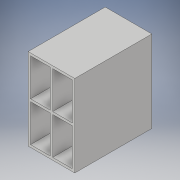
# Autodesk Inventor part: batterycart skeleton
Saved by Autodesk Inventor 2019 (Build 230136000, 136)
## iProperties
Created: 2018-12-03
Part Number: batterycart skeleton
Material: Generic
Document SubType Name: Modeling
Designer: Tiberus
Density: 1 g/cm^3
Appearance: Default
Author: Tiberus
Autodesk Inventor part; units mm, degrees
ref_plane "YZ Plane" through (0, 0, 0) normal (1, 0, 0) x (0, 1, 0)
ref_plane "XZ Plane" through (0, 0, 0) normal (0, 1, 0) x (-1, 0, 0)
ref_plane "XY Plane" through (0, 0, 0) normal (0, 0, 1) x (1, 0, 0)
sketch "Sketch1" plane through (0, 0, 0) normal (0, 0, 1) x (1, 0, 0)
  line L0 (0, 0) -> (241.3, 0)
  line L1 (241.3, 0) -> (241.3, 423.164)
  line L2 (241.3, 423.164) -> (0, 423.164)
  line L3 (0, 423.164) -> (0, 0)
  line L4 (120.65, 423.164) -> (120.65, 0) construction
  line L5 (241.3, 211.582) -> (0, 211.582) construction
  line L6 (159.3781, 211.582) -> (159.3781, 217.932) construction
  line L7 (120.65, 100.386) -> (127, 100.386) construction
  line L8 (196.0731, 0) -> (196.0731, 12.7) construction
  line L9 (142.6395, 423.164) -> (142.6395, 410.464) construction
  line L10 (127, 410.464) -> (228.6, 410.464)
  line L11 (127, 217.932) -> (228.6, 217.932)
  line L12 (228.6, 217.932) -> (228.6, 410.464)
  line L13 (241.3, 374.8885) -> (228.6, 374.8885) construction
  line L14 (174.8387, 211.582) -> (174.8387, 205.232) construction
  line L15 (127, 205.232) -> (228.6, 205.232)
  line L16 (228.6, 205.232) -> (228.6, 12.7)
  line L17 (228.6, 12.7) -> (127, 12.7)
  line L18 (127, 12.7) -> (127, 205.232)
  line L19 (127, 217.932) -> (127, 410.464)
  line L20 (81.9219, 211.582) -> (81.9219, 217.932) construction
  line L21 (114.3, 410.464) -> (12.7, 410.464)
  line L22 (114.3, 217.932) -> (12.7, 217.932)
  line L23 (12.7, 217.932) -> (12.7, 410.464)
  line L24 (66.4613, 211.582) -> (66.4613, 205.232) construction
  line L25 (114.3, 205.232) -> (12.7, 205.232)
  line L26 (12.7, 205.232) -> (12.7, 12.7)
  line L27 (12.7, 12.7) -> (114.3, 12.7)
  line L28 (114.3, 12.7) -> (114.3, 205.232)
  line L29 (114.3, 217.932) -> (114.3, 410.464)
  line L30 (120.65, 348.5591) -> (127, 348.5591) construction
  line L31 (228.6, 292.3608) -> (241.3, 292.3608) construction
  point P0 (45.2269, 12.7)
  point P1 (98.6605, 410.464)
  point P2 (12.7, 374.8885)
  dimension "d0" = 241.3
  dimension "d1" = 423.164
  dimension "d2" = 6.35
  dimension "d3" = 6.35
  dimension "d4" = 12.7
  dimension "d5" = 12.7
  dimension "d7" = 12.7
  dimension "d8" = 6.35
  dimension "d9" = 6.35
  dimension "d10" = 12.7
  constraints: 64 end point, 15 symmetric about line, 10 perpendicular, 10 point on line, 5 vertical, 4 horizontal, 4 midpoint, 2 parallel
  measures "d0" distance of L2.end L1.end
  measures "d1" distance of L1.end L0.end
  measures "d2" distance of L6.start L6.end
  measures "d3" distance of L7.start L7.end
  measures "d4" distance of L8.start L8.end
  measures "d5" distance of L9.start L9.end
  measures "d7" distance of L13.start L13.end
  measures "d8" distance of L14.start L14.end
  measures "d9" distance of L30.start L30.end
  measures "d10" distance of L31.start L31.end
extrude "Extrusion1" add sketch "Sketch1" along normal blind 398.78
sketch "Sketch2" plane through (241.3, 0, 0) normal (1, 0, 0) x (0, 0, -1)
  line L0 (0, 423.164) -> (-398.78, 423.164) construction
  line L1 (-199.39, 423.164) -> (-199.39, 0) construction
  line L2 (-199.39, 394.9054) -> (-193.04, 394.9054) construction
  line L3 (0, 0) -> (-398.78, 0) projected
  line L4 (-193.04, 0) -> (-193.04, 423.164)
  line L5 (-205.74, 0) -> (-205.74, 423.164)
  line L6 (-205.74, 0) -> (-193.04, 0)
  line L7 (-205.74, 423.164) -> (-193.04, 423.164)
  dimension "d13" = 6.35
  constraints: 12 end point, 3 point on line, 2 horizontal, 2 symmetric about line, 1 collinear, 1 midpoint, 1 perpendicular, 1 vertical
  measures "d13" distance of L2.start L2.end
extrude "Extrusion2" add sketch "Sketch2" against normal blind 241.3
body "Solid1"
